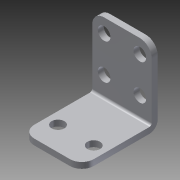
# Autodesk Inventor part: V5 Shooter Frame Channel Bracket Part 3
Saved by Autodesk Inventor 2014 SP1 (Build 180222100, 222)
## iProperties
Created: 2012-02-01
Part Number: V5 Shooter Frame Channel Bracket Part 3
Material: Aluminum-6061
Document SubType Name: Sheet Metal
Designer: Moses
Density: 2.71 g/cm^3
Sheet Metal Rule: Default
Mass: 18.7497 g
Surface Area: 54.1537 cm^2
Volume: 6.91871 cm^3
Flat Pattern Width: 3.175 cm
Flat Pattern Length: 7.62 cm
Flat Pattern Area: 24.1935 cm^2
Sheet Metal Width: 1.250 in
Sheet Metal Length: 3.000 in
Sheet Metal Area: 3.750 in^2
Appearance: Aluminum - Flat
Author: Moses
Autodesk Inventor part; units mm, degrees
ref_plane "YZ Plane" through (0, 0, 0) normal (1, 0, 0) x (0, 1, 0)
ref_plane "XZ Plane" through (0, 0, 0) normal (0, 1, 0) x (-1, 0, 0)
ref_plane "XY Plane" through (0, 0, 0) normal (0, 0, 1) x (1, 0, 0)
sketch "Sketch1" plane through (0, 0, 0) normal (0, 0, 1) x (1, 0, 0)
  line L0 (0, 0) -> (31.75, 0) construction
  line L1 (31.75, 0) -> (31.75, 38.1)
  line L2 (31.75, 38.1) -> (0, 38.1)
  line L3 (0, 38.1) -> (0, 0)
  line L4 (0, 0) -> (0, -38.1)
  line L5 (0, -38.1) -> (31.75, -38.1)
  line L6 (31.75, -38.1) -> (31.75, 0)
  line L7 (0, -25.4) -> (31.75, -25.4) construction
  circle A0 centre (25.4, -25.4) radius 3.3782
  line L8 (-19.05, -25.4) -> (12.7, -25.4) construction
  circle A1 centre (6.35, -25.4) radius 3.3782
  line L9 (0, -6.35) -> (31.75, -6.35) construction
  circle A2 centre (25.4, -6.35) radius 3.3782
  line L10 (-19.05, -6.35) -> (12.7, -6.35) construction
  circle A3 centre (6.35, -6.35) radius 3.3782
  line L11 (9.525, 1.27) -> (22.225, 1.27)
  line L12 (22.225, 1.27) -> (22.225, -1.27)
  line L13 (22.225, -1.27) -> (9.525, -1.27)
  line L14 (9.525, -1.27) -> (9.525, 1.27)
  point P0 (9.525, 0)
  dimension "d0" = 31.75
  dimension "d7" = 38.1
  dimension "d8" = 38.1
  dimension "d26" = 12.7
  dimension "d28" = 6.7564
  dimension "d30" = 6.35
  dimension "d33" = 19.05
  dimension "d36" = 19.05
  dimension "d52" = 12.7
  dimension "d53" = 2.54
  dimension "d54" = 9.525
  dimension "d55" = 31.75
  constraints: 30 end point, 7 point on line, 4 centre point, 4 parallel, 4 perpendicular, 3 vertical, 2 horizontal, 1 midpoint, 15 other
  measures "d0" distance of L0.start L0.end
  measures "d7" distance between parallel lines of L0 L2
  measures "d8" distance of L0.start L4.end
  measures "d26" distance between parallel lines of L5 L7
  measures "d28" diameter of A0
  measures "d30" distance from line of L6 A0.centre
  measures "d33" distance of L7.start L8.start
  measures "d36" distance of L7.start L9.start
  measures "d52" distance of L11.start L11.end
  measures "d53" distance of L11.end L12.end
  measures "d54" distance between parallel lines of L3 L14
  measures "d55" distance of L1.end L2.end
extrude "Plate1" add sketch "Sketch1" along normal blind 3.175 contours L6 L5 L4 L3 L2 L1 | A2 | A3 | L11 L12 L13 L14
fold "Fold1" angle 90 bend radius 1.27 thickness 3.175 k factor 0.44 line from (0, 0, 0) to (31.75, 0, 0) line at bend centre moving side (0, -1, 0) folds toward (0, 0, 1)
fillet "Corner Round1" radius 6.35 4 edges at (0, 38.1, 1.5875) (31.75, 38.1, 1.5875) (31.75, -0.7628, 40.4503) (0, -0.7628, 40.4503)
sketch "Sketch2" plane through (0, 0, 0) normal (0, 0, -1) x (-1, 0, 0)
  line L0 (-31.75, 31.75) -> (-31.75, 2.0947) projected
  line L1 (-31.75, 2.0947) -> (0, 2.0947) projected
  line L2 (-6.35, 38.1) -> (-25.4, 38.1) projected
  line L3 (0, -2.3503) -> (-31.75, -2.3503) construction
  circle A0 centre (-25.4, 30.6697) radius 3.3782
  circle A1 centre (-6.35, 30.6697) radius 3.3782
  circle A2 centre (-25.4, 11.6197) radius 3.3782
  circle A3 centre (-6.35, 11.6197) radius 3.3782
  line L4 (-25.4, 30.6697) -> (-6.35, 30.6697) construction
  line L5 (-15.875, 30.6697) -> (-15.875, 2.0947) construction
  point P0 (0, 0)
  dimension "d42" = 19.05
  dimension "d45" = 19.05
  dimension "d48" = 6.7564
  dimension "d49" = 13.97
  constraints: 4 centre point, 4 end point, 2 midpoint, 2 vertical, 1 horizontal, 1 parallel, 6 other
  measures "d42" distance of L4.start L4.end
  measures "d45" distance of L4.start A2.centre
  measures "d48" diameter of A0
  measures "d49" distance from line of L3 A3.centre
extrude "Cut1" cut sketch "Sketch2" against normal blind 3.175
equation "\"d28\" = d3"
equation "\"d30\" = -0.5 * d22 + 0.5 * d0"
equation "\"d33\" = d22"
equation "\"d36\" = d22"
equation "\"d10\" = BendReliefWidth"
equation "\"d11\" = BendReliefDepth"
equation "\"d12\" = MinimumRemnant"
equation "\"d13\" = BendRadius"
equation "\"d42\" = p1holespacing"
equation "\"d45\" = p1holespacing"
equation "\"d48\" = p1mountholedia"
equation "\"d49\" = p1holedistedge"
equation "\"d50\" = Thickness"
equation "\"BendRadius\" = Thickness"
equation "\"BendReliefWidth\" = Thickness"
equation "\"BendReliefDepth\" = 0.5 * Thickness"
equation "\"CornerReliefSize\" = 4 * Thickness"
equation "\"MinimumRemnant\" = 2 * Thickness"
equation "\"TransitionRadius\" = BendRadius"
equation "\"JacobiRadiusSize\" = BendRadius"
equation "\"GapSize\" = Thickness"
equation "\"d3\" = d4"
equation "\"d4\" = p1mountholedia"
equation "\"d9\" = BendRadius"
equation "\"d22\" = p1holespacing"
equation "\"p1holespacing\" = 19.05"
equation "\"p1mountholedia\" = 6.7564"
equation "\"p1holedistedge\" = 13.97"
equation "\"Thickness\" = 3.175"
body "Solid1"
